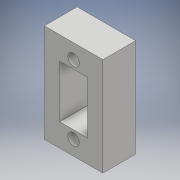
# Autodesk Inventor part: slot złącze
Saved by Autodesk Inventor 2017 (Build 210142000, 142)
## iProperties
Created: 2019-10-08
Part Number: slot złącze
Material: Ogólny
Document SubType Name: Modeling
Designer: patry
Density: 1 g/cm^3
Appearance: Domyślna
Author: patry
Autodesk Inventor part; units mm, degrees
ref_plane "YZ Plane" through (0, 0, 0) normal (1, 0, 0) x (0, 1, 0)
ref_plane "XZ Plane" through (0, 0, 0) normal (0, 1, 0) x (-1, 0, 0)
ref_plane "XY Plane" through (0, 0, 0) normal (0, 0, 1) x (1, 0, 0)
sketch "Szkic1" plane through (0, 0, 0) normal (0, 1, 0) x (-1, 0, 0)
  line L0 (-4.25, 8) -> (4.25, 8)
  line L1 (4.25, 8) -> (4.25, -8)
  line L2 (4.25, -8) -> (-4.25, -8)
  line L3 (-4.25, -8) -> (-4.25, 8)
  line L4 (-4.25, 8) -> (4.25, -8) construction
  line L5 (4.25, 8) -> (-4.25, -8) construction
  circle A0 centre (0, -10.5) radius 1.75
  circle A1 centre (0, 10.5) radius 1.75
  line L6 (-8.9265, 15) -> (8.9265, 15)
  line L7 (8.9265, 15) -> (8.9265, -15)
  line L8 (8.9265, -15) -> (-8.9265, -15)
  line L9 (-8.9265, -15) -> (-8.9265, 15)
  line L10 (-8.9265, 15) -> (8.9265, -15) construction
  line L11 (8.9265, 15) -> (-8.9265, -15) construction
  point P0 (0, 0)
  dimension "d0" = 8.5
  dimension "d1" = 16
  dimension "d2" = 3.5
  dimension "d3" = 4.25
  dimension "d4" = 10.5
  dimension "d5" = 3.5
  dimension "d6" = 4.25
  dimension "d7" = 10.5
  constraints: 24 end point, 4 midpoint, 4 parallel, 2 centre point, 2 horizontal, 2 perpendicular
  measures "d0" distance of L1.end L2.end
  measures "d1" distance of L0.end L1.end
  measures "d2" diameter of A0
  measures "d3" distance from line of A0.centre L1
  measures "d4" distance of point (0, 0) A0.centre
  measures "d5" diameter of A1
  measures "d6" distance from line of L1 A1.centre
  measures "d7" distance of point (0, 0) A1.centre
extrude "Wyciągnięcie proste1" add sketch "Szkic1" along normal blind 10
equation "\"d3\" = 0.5 * d0"
equation "\"d5\" = d2"
equation "\"d6\" = d3"
equation "\"d7\" = d4"
